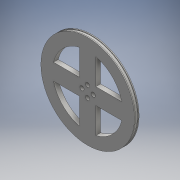
# Autodesk Inventor part: wheel
Saved by Autodesk Inventor 2016 (Build 200138000, 138)
## iProperties
Created: 2016-02-18
Part Number: wheel
Material: Generic
Document SubType Name: Modeling
Designer: mkepler
Density: 1 g/cm^3
Appearance: Default
Author: mkepler
Autodesk Inventor part; units mm, degrees
ref_plane "YZ Plane" through (0, 0, 0) normal (1, 0, 0) x (0, 1, 0)
ref_plane "XZ Plane" through (0, 0, 0) normal (0, 1, 0) x (-1, 0, 0)
ref_plane "XY Plane" through (0, 0, 0) normal (0, 0, 1) x (1, 0, 0)
sketch "Sketch1" plane through (0, 0, 0) normal (0, 1, 0) x (-1, 0, 0)
  circle A0 centre (0, 0) radius 50
  circle A1 centre (0, 0) radius 37.5
  circle A2 centre (0, 0) radius 8.75
  line L0 (37.5, 0) -> (42.141, 0) construction
  line L1 (8.75, -8.75) -> (36.4649, -8.75)
  line L2 (-8.75, -8.75) -> (-36.4649, -8.75)
  line L3 (-8.75, -8.75) -> (-8.75, -36.4649)
  line L4 (8.75, -8.75) -> (8.75, -36.4649)
  line L5 (8.75, 8.75) -> (36.4649, 8.75)
  line L6 (-8.75, 8.75) -> (-36.4649, 8.75)
  line L7 (-8.75, 8.75) -> (-8.75, 36.4649)
  line L8 (8.75, 8.75) -> (8.75, 36.4649)
  dimension "d1" = 75
  dimension "d0" = 100
  dimension "d2" = 17.5
  constraints: 18 end point, 3 coincident, 3 horizontal, 2 centre point, 2 perpendicular, 2 tangent, 1 parallel, 1 point on line, 11 other
  measures "d0" diameter of A0
  measures "d2" diameter of A2
extrude "Extrusion1" add sketch "Sketch1" along normal blind 1 contours A0 | A1 L1 L4 L3 L2 L6 L7 L8 L5 | A2
sketch "Sketch6" plane through (0, 1, 0) normal (0, 1, 0) x (1, 0, 0)
  circle A0 centre (0, 0) radius 49.25
  line L0 (-36.4649, -8.75) -> (-8.75, -8.75) projected
  line L1 (-8.6444, -8.75) -> (-36.4649, -8.75)
  arc A1 (-36.4649, -8.75) -> (-8.75, -36.4649) centre (0, 0) ccw projected
  line L2 (-36.4649, -8.75) -> (-36.4649, -8.75)
  line L3 (-8.75, -36.4649) -> (-8.75, -8.75) projected
  line L4 (-8.75, -8.75) -> (-8.75, -36.4649)
  arc A2 (-36.4649, -8.75) -> (-8.75, -36.4649) centre (0, 0) ccw
  line L5 (0, 0) -> (0, -21.0072)
  line L6 (0, 0) -> (-15.0352, 0)
  line L7 (36.4649, -8.75) -> (8.75, -8.75)
  arc A3 (8.75, -36.4649) -> (36.4649, -8.75) centre (0, 0) ccw
  line L8 (8.75, -36.4649) -> (8.75, -8.75)
  line L9 (-36.4649, 8.75) -> (-8.75, 8.75)
  arc A4 (-8.75, 36.4649) -> (-36.4649, 8.75) centre (0, 0) ccw
  line L10 (-8.75, 36.4649) -> (-8.75, 8.75)
  arc A5 (36.4649, 8.75) -> (8.75, 36.4649) centre (0, 0) ccw
  line L11 (36.4649, 8.75) -> (8.75, 8.75)
  line L12 (8.75, 36.4649) -> (8.75, 8.75)
  dimension "d33" = 98.5
  constraints: 22 end point, 9 symmetric about line, 8 point on circle, 5 centre point, 2 collinear, 1 coincident, 1 concentric, 1 horizontal, 1 vertical, 3 other
  measures "d33" diameter of A0
extrude "Extrusion3" add sketch "Sketch6" along normal blind 3
sketch "Sketch7" plane through (0, 4, 0) normal (0, 1, 0) x (1, 0, 0)
  circle A0 centre (0, 0) radius 50
  line L0 (-8.75, -36.4649) -> (-8.75, -8.75) projected
  arc A1 (-36.4649, -8.75) -> (-8.75, -36.4649) centre (0, 0) ccw projected
  line L1 (-8.75, -8.75) -> (-36.4649, -8.75)
  line L2 (-8.75, -8.75) -> (-8.75, -36.4649)
  arc A2 (-36.4649, -8.75) -> (-8.75, -36.4649) centre (0, 0) ccw
  line L3 (0, 0) -> (0, -13.8921)
  line L4 (0, 0) -> (-12.1262, 0)
  line L5 (8.75, -36.4649) -> (8.75, -8.75)
  arc A3 (8.75, -36.4649) -> (36.4649, -8.75) centre (0, 0) ccw
  line L6 (8.75, -8.75) -> (36.4649, -8.75)
  line L7 (-8.75, 36.4649) -> (-8.75, 8.75)
  arc A4 (-8.75, 36.4649) -> (-36.4649, 8.75) centre (0, 0) ccw
  line L8 (-8.75, 8.75) -> (-36.4649, 8.75)
  line L9 (8.75, 8.75) -> (36.4649, 8.75)
  arc A5 (36.4649, 8.75) -> (8.75, 36.4649) centre (0, 0) ccw
  line L10 (8.75, 36.4649) -> (8.75, 8.75)
  dimension "d37" = 100
  constraints: 20 end point, 9 point on circle, 9 symmetric about line, 5 centre point, 2 horizontal, 1 coincident, 1 concentric, 1 vertical, 3 other
  measures "d37" diameter of A0
extrude "Extrusion4" add sketch "Sketch7" along normal blind 1
sketch "Sketch8" plane through (0, 5, 0) normal (0, 1, 0) x (1, 0, 0)
  circle A0 centre (0, 6) radius 2.25
  line L0 (0, 0) -> (-6, 0)
  line L1 (0, 0) -> (0, -5.6539)
  circle A1 centre (0, -6) radius 2.25
  circle A2 centre (-6, 0) radius 2.25
  circle A3 centre (6, 0) radius 2.25
  dimension "d40" = 4.5
  dimension "d41" = 6
  dimension "d42" = 4.5
  dimension "d43" = 6
  constraints: 4 centre point, 4 end point, 3 symmetric about line, 2 coincident, 1 horizontal, 1 vertical, 2 other
  measures "d40" diameter of A0
  measures "d41" distance of A0.centre L0.start
  measures "d42" diameter of A2
  measures "d43" distance of L0.start L0.end
hole "Hole2" at (0, 5, 6) at (-6, 5, 0) at (0, 5, -6) at (6, 5, 0) direction (0, -1, 0) diameter 4.5 end through all
body "Solid1"
